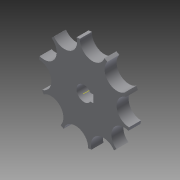
# Autodesk Inventor part: gear
Saved by Autodesk Inventor 2015 (Build 190159000, 159)
## iProperties
Created: 2016-03-12
Part Number: gear
Material: Generic
Document SubType Name: Modeling
Designer: clopez42
Density: 1 g/cm^3
Appearance: Default
Author: clopez42
Autodesk Inventor part; units mm, degrees
ref_plane "YZ Plane" through (0, 0, 0) normal (1, 0, 0) x (0, 1, 0)
ref_plane "XZ Plane" through (0, 0, 0) normal (0, 1, 0) x (-1, 0, 0)
ref_plane "XY Plane" through (0, 0, 0) normal (0, 0, 1) x (1, 0, 0)
sketch "Sketch1" plane through (0, 0, 0) normal (0, 1, 0) x (-1, 0, 0)
  arc A0 (-5.3837, -3.1747) -> (-5.3833, 3.1753) centre (0, 0) ccw
  line L0 (-5.3833, 3.1753) -> (-7.8217, 3.1753)
  line L1 (-5.3837, -3.1747) -> (-7.8217, -3.1747)
  line L2 (-7.8217, 3.1753) -> (-7.8217, -3.1747)
  circle A1 centre (0, 0) radius 27.5 construction
  circle A2 centre (0, 0) radius 38
  arc A3 (37.5726, 5.6835) -> (34.9367, -14.9474) centre (37.6936, -4.8158) ccw
  arc A4 (27.0562, 26.6827) -> (37.0503, 8.4426) centre (33.3254, 18.2597) ccw
  arc A5 (6.2052, 37.4899) -> (25.0119, 28.6078) centre (16.228, 34.3606) ccw
  arc A6 (-17.0159, 33.9773) -> (3.4198, 37.8458) centre (-7.0679, 37.3369) ccw
  arc A7 (-33.7375, 17.4865) -> (-19.4786, 32.628) centre (-27.6641, 26.0518) ccw
  arc A8 (-37.5726, -5.6835) -> (-34.9367, 14.9474) centre (-37.6936, 4.8158) ccw
  arc A9 (-27.0562, -26.6827) -> (-37.0503, -8.4426) centre (-33.3254, -18.2597) ccw
  arc A10 (-6.2052, -37.4899) -> (-25.0119, -28.6078) centre (-16.228, -34.3606) ccw
  arc A11 (17.0159, -33.9773) -> (-3.4198, -37.8458) centre (7.0679, -37.3369) ccw
  arc A12 (33.7375, -17.4865) -> (19.4786, -32.628) centre (27.6641, -26.0518) ccw
  dimension "d0" = 12.5
  dimension "d1" = 6.35
  dimension "d2" = 2.4384
  dimension "d3" = 2.438
  dimension "d4" = 55
  dimension "d5" = 76
  dimension "d6" = 10.5
  dimension "d9" = 360
  constraints: 24 point on circle, 13 centre point, 6 end point, 3 coincident, 2 horizontal, 1 tangent, 1 vertical, 41 other
  measures "d0" diameter of A0
  measures "d1" distance of L0.end L1.end
  measures "d2" distance of L0.start L0.end
  measures "d3" distance of L1.start L1.end
  measures "d4" diameter of A1
  measures "d5" diameter of A2
  measures "d6" radius of A3
extrude "Extrusion1" add sketch "Sketch1" along normal blind 10 contours A3 A2 A12 A11 A10 A9 A8 A7 A6 A5 A4 | A4 A2 | A2 A12 | A5 A2 | A2 A11 | A6 A2 | A2 A10 | A7 A2 | A2 A9 | A8 A2
sketch "Sketch2" plane through (0, 10, 0) normal (0, 1, 0) x (1, 0, 0)
  arc A0 (-37.5726, -5.6835) -> (-34.9367, 14.9474) centre (-37.6936, 4.8158) ccw projected
  arc A1 (-37.5726, -5.6835) -> (-34.9367, 14.9474) centre (-37.6936, 4.8158) ccw projected
  circle A2 centre (0, 0) radius 38 projected
  arc A3 (-27.0562, -26.6827) -> (-37.0503, -8.4426) centre (-33.3254, -18.2597) ccw projected
hole "Hole1" at (-33.3254, 10, 18.2597) direction (0, -1, 0) diameter 21 end through all
pattern_circular "Circular Pattern1" count 10 over 360 about axis through (0, 10, 0) along (0, -1, 0) of "Hole1"
body "Solid1"
